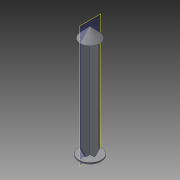
# Autodesk Inventor part: syringe inner
Saved by Autodesk Inventor 2015 SP1 (Build 190203100, 203)
## iProperties
Created: 2016-07-08
Part Number: syringe inner
Material: Generic
Document SubType Name: Modeling
Designer: lustinga
Density: 1 g/cm^3
Appearance: Default
Mass: 19.3037 g
Surface Area: 168.045 cm^2
Volume: 19.3037 cm^3
Author: lustinga
Autodesk Inventor part; units mm, degrees
ref_plane "YZ Plane" through (0, 0, 0) normal (1, 0, 0) x (0, 1, 0)
ref_plane "XZ Plane" through (0, 0, 0) normal (0, 1, 0) x (-1, 0, 0)
ref_plane "XY Plane" through (0, 0, 0) normal (0, 0, 1) x (1, 0, 0)
sketch "Sketch1" plane through (0, 0, 0) normal (0, 0, 1) x (1, 0, 0)
  line L0 (3.9669, 12.6467) -> (5.1169, 12.6467)
  line L1 (5.1169, 12.6467) -> (5.1169, 1.1467)
  line L2 (5.1169, 1.1467) -> (16.6169, 1.1467)
  line L3 (16.6169, 1.1467) -> (16.6169, -1.1533)
  line L4 (16.6169, -1.1533) -> (5.1169, -1.1533)
  line L5 (5.1169, -1.1533) -> (5.1169, -12.6533)
  line L6 (5.1169, -12.6533) -> (3.9669, -12.6533)
  line L7 (3.9669, 12.6467) -> (2.8169, 12.6467)
  line L8 (2.8169, 12.6467) -> (2.8169, 1.1467)
  line L9 (2.8169, 1.1467) -> (-8.6831, 1.1467)
  line L10 (-8.6831, 1.1467) -> (-8.6831, -1.1533)
  line L11 (-8.6831, -1.1533) -> (2.8169, -1.1533)
  line L12 (2.8169, -1.1533) -> (2.8169, -12.6533)
  line L13 (2.8169, -12.6533) -> (3.9669, -12.6533)
  point P0 (0, 0)
  dimension "d0" = 1.15
  dimension "d1" = 2.3
  dimension "d2" = 11.5
  dimension "d3" = 11.5
  dimension "d4" = 11.5
  dimension "d5" = 11.5
  dimension "d6" = 1.15
  constraints: 28 end point, 6 perpendicular, 1 horizontal
  measures "d0" distance of L0.start L0.end
  measures "d1" distance of L2.end L3.end
  measures "d2" distance of L0.end L1.end
  measures "d3" distance of L1.end L2.end
  measures "d4" distance of L3.end L4.end
  measures "d5" distance of L4.end L5.end
  measures "d6" distance of L5.end L6.end
extrude "Extrusion1" add sketch "Sketch1" along normal blind 140
ref_plane "Work Plane1" through (3.9669, 1.1467, 0) normal (-1, 0, 0) x (0, 0, 1)
sketch "Sketch4" plane through (3.9669, 1.1467, 0) normal (-1, 0, 0) x (0, 0, 1)
  line L0 (3.9669, 12.6467) -> (5.1169, 12.6467)
  line L1 (5.1169, 12.6467) -> (5.1169, 1.1467)
  line L2 (5.1169, 1.1467) -> (16.6169, 1.1467)
  line L3 (16.6169, 1.1467) -> (16.6169, -1.1533)
  line L4 (16.6169, -1.1533) -> (5.1169, -1.1533)
  line L5 (5.1169, -1.1533) -> (5.1169, -12.6533)
  line L6 (5.1169, -12.6533) -> (3.9669, -12.6533)
  line L7 (2.8169, 12.6467) -> (2.8169, 1.1467)
  line L8 (2.8169, 1.1467) -> (-8.6831, 1.1467)
  line L9 (-8.6831, 1.1467) -> (-8.6831, -1.1533)
  line L10 (-8.6831, -1.1533) -> (2.8169, -1.1533)
  line L11 (2.8169, -1.1533) -> (2.8169, -12.6533)
  line L12 (2.8169, -12.6533) -> (3.9669, -12.6533)
  line L13 (3.9669, 12.6467) -> (2.8169, 12.6467)
  line L14 (140, -13.8) -> (140, 11.5) projected
  line L15 (140, -13.6427) -> (140, -13.8) projected
  line L16 (140, -2.3) -> (140, -13.6427) projected
  line L17 (140, 0) -> (140, -2.3) projected
  line L18 (140, 11.3427) -> (140, 0) projected
  line L19 (140, 11.5) -> (140, 11.3427) projected
  line L20 (154, -1.15) -> (140, 12.35)
  line L21 (140, 11.3427) -> (140, 0) projected
  line L22 (154, -1.15) -> (140, -1.15)
  line L23 (140, 12.35) -> (140, -1.15)
  line L24 (154.6806, -1.15) -> (155.8888, -1.15)
  point P0 (0, -1.1467)
  point P1 (0, 0)
  point P2 (154, -1.15)
  dimension "d13" = 1.15
  dimension "d14" = 2.3
  dimension "d15" = 11.5
  dimension "d16" = 11.5
  dimension "d17" = 11.5
  dimension "d18" = 11.5
  dimension "d19" = 1.15
  constraints: 36 end point, 6 perpendicular, 2 point on line, 1 coincident, 1 collinear, 1 horizontal, 1 midpoint
  measures "d13" distance of L0.start L0.end
  measures "d14" distance of L2.end L3.end
  measures "d15" distance of L0.end L1.end
  measures "d16" distance of L1.end L2.end
  measures "d17" distance of L3.end L4.end
  measures "d18" distance of L4.end L5.end
  measures "d19" distance of L5.end L6.end
revolve "Revolution2" add sketch "Sketch4" angle 360 about axis through (3.9669, -0.0033, 154.6806) along (0, 0, 1) contours L14 L23 L20 L22
sketch "Sketch5" plane through (0, 0, 0) normal (0, 0, -1) x (-1, 0, 0)
  circle A0 centre (-3.9669, -0.0033) radius 13.5 projected
  circle A1 centre (-3.9669, -0.0033) radius 15.45
  point P0 (0, 0)
  dimension "d21" = 30.9
  constraints: 1 centre point, 1 coincident
  measures "d21" diameter of A1
extrude "Extrusion2" add sketch "Sketch5" along normal blind 1.87 contours A0 | A1
sketch "Sketch6" plane through (3.9669, 1.1467, 0) normal (-1, 0, 0) x (0, 0, 1)
  line L0 (0, 11.5) -> (0, 0) projected
  line L1 (0, 11.5) -> (140, 11.5) projected
  line L2 (0, -1.1467) -> (5.329, -1.1467)
  line L3 (0, 14.3) -> (-1.87, 14.3) projected
  line L4 (0, 14.3) -> (0, 7.3)
  line L5 (0, 0) -> (0, 11.5) projected
  line L6 (0, 14.3) -> (18, 14.3)
  line L7 (18, 14.3) -> (0, 5.75)
  point P0 (0, 7.85)
  point P1 (12, 11.5)
  dimension "d27" = 7
  constraints: 8 end point, 3 point on line, 2 horizontal, 1 midpoint
  measures "d27" distance of L3.start L4.end
revolve "Revolution3" cut sketch "Sketch6" angle 360 about axis through (3.9669, 0, 0) along (0, 0, 1)
body "Solid1"
